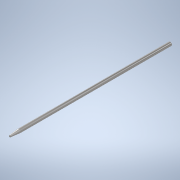
# Autodesk Inventor part: bolec
Saved by Autodesk Inventor 2021 (Build 250183000, 183)
## iProperties
Created: 2021-05-20
Part Number: bolec
Material: Stal nierdzewna
Document SubType Name: Modeling
Designer: Wojciech Wołczek
Density: 8 g/cm^3
Appearance: Częściowo polerowana
Author: Wojciech Wołczek
Autodesk Inventor part; units mm, degrees
ref_plane "YZ Plane" through (0, 0, 0) normal (1, 0, 0) x (0, 1, 0)
ref_plane "XZ Plane" through (0, 0, 0) normal (0, 1, 0) x (-1, 0, 0)
ref_plane "XY Plane" through (0, 0, 0) normal (0, 0, 1) x (1, 0, 0)
sketch "Szkic1" plane through (0, 0, 0) normal (0, 0, 1) x (1, 0, 0)
  circle A0 centre (0, 0) radius 2
  dimension "d0" = 4
  constraints: 1 centre point, 1 coincident
  measures "d0" diameter of A0
extrude "Wyciągnięcie proste1" add sketch "Szkic1" along normal blind 180
chamfer "Faza1" distance 1 distance2 10 1 edges at (-2, 0, 180) measured on face at (-1.5, 0, 180)
